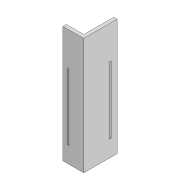
# Autodesk Inventor part: Knife_guide_30deg_20mm
Saved by Autodesk Inventor 2022 (Build 260153000, 153)
## iProperties
Created: 2022-06-30
Part Number: Knife_guide_30deg_20mm
Material: Generic
Document SubType Name: Modeling
Designer: dell
Density: 1 g/cm^3
Appearance: Default
Author: dell
Autodesk Inventor part; units mm, degrees
ref_plane "YZ Plane" through (0, 0, 0) normal (1, 0, 0) x (0, 1, 0)
ref_plane "XZ Plane" through (0, 0, 0) normal (0, 1, 0) x (-1, 0, 0)
ref_plane "XY Plane" through (0, 0, 0) normal (0, 0, 1) x (1, 0, 0)
sketch "Sketch1" plane through (0, 0, 0) normal (0, 1, 0) x (-1, 0, 0)
  line L0 (0, 0) -> (25, 0)
  line L1 (25, 0) -> (25, -40)
  line L2 (25, -40) -> (0, -40)
  line L3 (0, -40) -> (0, 0)
  line L4 (25, -40) -> (4, -40)
  line L5 (4, -40) -> (4, -4)
  line L6 (4, -4) -> (25, -4)
  line L7 (25, -4) -> (25, -40)
  point P0 (25, -4)
  dimension "d0" = 4
  dimension "d1" = 4
  dimension "d2" = 40
  dimension "d3" = 25
  constraints: 16 end point, 4 parallel, 2 horizontal, 2 perpendicular
  measures "d0" distance between parallel lines of L3 L5
  measures "d1" distance between parallel lines of L0 L6
  measures "d2" distance between parallel lines of L0 L2
  measures "d3" distance between parallel lines of L1 L3
extrude "Extrusion1" add sketch "Sketch1" along normal blind 100 contours L0 L1 L6 L5 L2 L3
sketch "Sketch2" plane through (0, 100, 0) normal (0, 1, 0) x (1, 0, 0)
  line L0 (0, 0) -> (0, 40) projected
  line L1 (0, 40) -> (-4, 40) projected
  line L2 (-4, 40) -> (-4, 4) projected
  line L3 (-4, 4) -> (-25, 4) projected
  line L4 (-25, 4) -> (-25, 0) projected
  line L5 (-25, 0) -> (0, 0) projected
  line L6 (-25, 0) -> (0, 0) projected
  line L7 (-17.8564, 0) -> (0, 30.9282)
  line L8 (0, 0) -> (0, 40) projected
  line L9 (0, 32.9282) -> (-19.0111, 0)
  line L10 (-4, 40) -> (-4, 4) projected
  point P0 (-16.7017, 4)
  point P1 (-19.0111, 0)
  point P2 (-17.8564, 0)
  point P3 (-15.547, 4)
  point P4 (0, 32.9282)
  point P5 (-4, 26)
  point P6 (-4, 24)
  point P7 (0, 30.9282)
  point P8 (-4, 24)
  dimension "d7" = 30
  dimension "d8" = 1
  dimension "d11" = 20
  constraints: 6 point on line, 4 end point, 1 parallel
  measures "d7" angle of L0 L7
  measures "d8" distance between parallel lines of L9 L7
  measures "d11" distance from line of L3 point (-4, 24)
extrude "Extrusion2" cut sketch "Sketch2" against normal blind 80 contours L7 L2 L9 L0 | L5 L9 L3 L7 | L7 L3 L9 L2
sketch "Sketch3" plane through (0, 100, 0) normal (0, 1, 0) x (1, 0, 0)
  line L0 (-19.0111, 0) -> (-16.7017, 4) projected
  line L1 (-16.7017, 4) -> (-25, 4) projected
  line L2 (-25, 4) -> (-25, 0) projected
  line L3 (-25, 0) -> (-19.0111, 0) projected
  line L4 (-15.547, 4) -> (-17.8564, 0) projected
  line L5 (-17.8564, 0) -> (0, 0) projected
  line L6 (0, 0) -> (0, 30.9282) projected
  line L7 (0, 30.9282) -> (-4, 24) projected
  line L8 (-4, 24) -> (-4, 4) projected
  line L9 (-4, 4) -> (-15.547, 4) projected
  line L10 (-4, 26) -> (0, 32.9282) projected
  line L11 (0, 32.9282) -> (0, 40) projected
  line L12 (0, 40) -> (-4, 40) projected
  line L13 (-4, 40) -> (-4, 26) projected
  line L14 (-16.7017, 4) -> (-15.547, 4) projected
  line L15 (-19.0111, 0) -> (-16.7017, 4) projected
  line L16 (-17.8564, 0) -> (-19.0111, 0) projected
  line L17 (-15.547, 4) -> (-17.8564, 0) projected
  line L18 (-4, 24) -> (-4, 26) projected
  line L19 (0, 30.9282) -> (-4, 24) projected
  line L20 (0, 32.9282) -> (0, 30.9282) projected
  line L21 (-4, 26) -> (0, 32.9282) projected
  point P0 (0, 32.9282)
extrude "Extrusion3" add sketch "Sketch3" along normal blind 40
body "Solid1"
